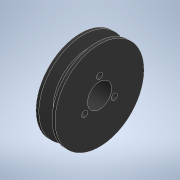
# Autodesk Inventor part: Pulley - VBelt (2.5in OD)
Saved by Autodesk Inventor 2022.1 (Build 261234020, 234B)
## iProperties
Created: 2022-04-06
Part Number: Pulley - VBelt (2.5in OD)
Material: Nylon 6/6
Document SubType Name: Modeling
Designer: NCai2
Density: 1.13 g/cm^3
Appearance: Rubber - Black
Mass: 6.74484 g
Surface Area: 44.5721 cm^2
Volume: 5.96888 cm^3
Author: NCai2
Autodesk Inventor part; units mm, degrees
ref_plane "YZ Plane" through (0, 0, 0) normal (1, 0, 0) x (0, 1, 0)
ref_plane "XZ Plane" through (0, 0, 0) normal (0, 1, 0) x (-1, 0, 0)
ref_plane "XY Plane" through (0, 0, 0) normal (0, 0, 1) x (1, 0, 0)
sketch "Sketch1" plane through (0, 0, 0) normal (0, 0, 1) x (1, 0, 0)
  line L0 (0, 0) -> (4.7625, 0) construction
  line L1 (4.7625, 0) -> (4.7625, 22.225)
  line L2 (4.7625, 22.225) -> (0, 22.225)
  line L3 (0, 22.225) -> (0, 0)
  line L4 (3.3, 22.225) -> (1.4923, 16.975)
  line L5 (1.4923, 16.975) -> (0, 16.975)
  line L6 (0, 6) -> (4.7625, 6)
  line L7 (0, 0) -> (-4.7625, 0) construction
  line L8 (-4.7625, 0) -> (-4.7625, 22.225)
  line L9 (-4.7625, 22.225) -> (0, 22.225)
  line L10 (-3.3, 22.225) -> (-1.4923, 16.975)
  line L11 (-1.4923, 16.975) -> (0, 16.975)
  line L12 (0, 6) -> (-4.7625, 6)
  dimension "d0" = 4.7625
  dimension "d1" = 22.225
  dimension "d2" = 19
  dimension "d3" = 3.3
  dimension "d4" = 5.25
  dimension "d5" = 6
  constraints: 26 end point, 6 point on line, 5 symmetric about line, 3 perpendicular, 2 parallel, 1 horizontal
  measures "d0" distance of L2.end L1.end
  measures "d1" distance of L1.end L0.end
  measures "d2" angle of L3 L4
  measures "d3" distance of L2.end L4.start
  measures "d4" distance between parallel lines of L2 L5
  measures "d5" distance between parallel lines of L0 L6
revolve "Revolution1" add sketch "Sketch1" angle 360 about axis through (0, 0, 0) along (-1, 0, 0) contours L6 L3 L5 L4 L2 L1 | L12 L8 L9 L10 L11 L3
sketch "Sketch4" plane through (4.7625, 0, 0) normal (1, 0, 0) x (0, 0, -1)
  circle A0 centre (0, 8.5) radius 1.5
  circle A1 centre (-7.3612, -4.25) radius 1.5
  circle A2 centre (7.3612, -4.25) radius 1.5
  point P0 (0, 0)
  dimension "d40" = 3
  dimension "d41" = 8.5
  dimension "d44" = 360
  constraints: 3 centre point, 7 other
  measures "d40" diameter of A0
  measures "d41" distance of point (0, 0) A0.centre
extrude "Extrusion3" cut sketch "Sketch4" against normal through all
body "Solid1"
